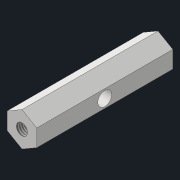
# Autodesk Inventor part: pistony
Saved by Autodesk Inventor 2022 (Build 260153000, 153)
## iProperties
Created: 2022-09-22
Part Number: pistony
Material: Generic
Document SubType Name: Modeling
Designer: Kieran Jarvis
Density: 1 g/cm^3
Appearance: Default
Author: Kieran Jarvis
Autodesk Inventor part; units mm, degrees
ref_plane "YZ Plane" through (0, 0, 0) normal (1, 0, 0) x (0, 1, 0)
ref_plane "XZ Plane" through (0, 0, 0) normal (0, 1, 0) x (-1, 0, 0)
ref_plane "XY Plane" through (0, 0, 0) normal (0, 0, 1) x (1, 0, 0)
sketch "Sketch1" plane through (0, 0, 0) normal (0, 0, 1) x (1, 0, 0)
  line L0 (0, -7.3323) -> (-6.35, -3.6662)
  line L1 (-6.35, -3.6662) -> (-6.35, 3.6662)
  line L2 (-6.35, 3.6662) -> (0, 7.3323)
  line L3 (0, 7.3323) -> (6.35, 3.6662)
  line L4 (6.35, 3.6662) -> (6.35, -3.6662)
  line L5 (6.35, -3.6662) -> (0, -7.3323)
  circle A0 centre (0, 0) radius 3
  dimension "d0" = 12.7
  dimension "d1" = 6
  constraints: 12 end point, 2 coincident, 1 centre point, 1 vertical, 13 other
  measures "d0" distance between parallel lines of L3 L0
  measures "d1" diameter of A0
extrude "Extrusion2" add sketch "Sketch1" along normal mid plane 58.5 contours L0 L1 L2 L3 L4 L5 | A0
sketch "Sketch4" plane through (-6.35, -3.6662, -29.25) normal (-1, 0, 0) x (0, 0, 1)
  line L0 (58.5, 7.3323) -> (58.5, 0) projected
  line L1 (0, 0) -> (0, 7.3323) projected
  point P0 (29.25, 3.6662)
  point P1 (29.25, 3.6662)
  point P2 (58.5, 3.6662)
  dimension "d43" = 58.5
  constraints: 1 coincident, 1 horizontal alignment, 1 midpoint
  measures "d43" distance between parallel lines of L1 L0
hole "Hole4" at (-6.35, 0, 0) direction (1, 0, 0) diameter 6 end through all
sketch "Sketch5" plane through (0, 0, -29.25) normal (0, 0, -1) x (-1, 0, 0)
  point P0 (0, 0)
  point P1 (0, 0)
  constraints: 1 coincident
hole "Hole5" at (0, 0, -29.25) direction (0, 0, 1) diameter 4.917 depth 17.1 tip angle 118 thread size "M6x1" class "6H" standard "ISO Metric profile"
mirror "Mirror1" about plane through (0, 0, 0) normal (0, 0, 1) of "Hole5"
body "Solid2"
